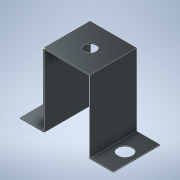
# Autodesk Inventor part: cla3
Saved by Autodesk Inventor 2021 (Build 250183000, 183)
## iProperties
Created: 2021-07-06
Part Number: cla3
Material: Iron, Cast
Document SubType Name: Modeling
Designer: KAVYA
Density: 7.15 g/cm^3
Appearance: Iron Gray
Author: KAVYA
Autodesk Inventor part; units mm, degrees
ref_plane "YZ Plane" through (0, 0, 0) normal (1, 0, 0) x (0, 1, 0)
ref_plane "XZ Plane" through (0, 0, 0) normal (0, 1, 0) x (-1, 0, 0)
ref_plane "XY Plane" through (0, 0, 0) normal (0, 0, 1) x (1, 0, 0)
sketch "Sketch1" plane through (0, 0, 0) normal (0, 1, 0) x (-1, 0, 0)
  line L0 (0, 0) -> (-48, 0)
  line L1 (-48, 0) -> (-48, -50)
  line L2 (-48, -50) -> (0, -50)
  line L3 (0, -50) -> (0, 0)
  dimension "d0" = 48
  dimension "d1" = 50
  constraints: 8 end point, 2 parallel, 1 horizontal, 1 perpendicular
  measures "d0" distance of L2.end L1.end
  measures "d1" distance of L1.end L0.end
extrude "Extrusion1" add sketch "Sketch1" along normal blind 1
sketch "Sketch2" plane through (48, 0, 0) normal (1, 0, 0) x (0, 0, -1)
  line L0 (0, 1) -> (50, 1) projected
  line L1 (0, 1) -> (50, 1)
  line L2 (50, 1) -> (50, -76)
  line L3 (50, -76) -> (0, -76)
  line L4 (0, -76) -> (0, 1)
  point P0 (0, 0)
  dimension "d4" = 50
  dimension "d5" = 77
  constraints: 8 end point, 2 parallel, 1 horizontal, 1 perpendicular
  measures "d4" distance of L2.end L3.end
  measures "d5" distance of L1.end L2.end
extrude "Extrusion2" add sketch "Sketch2" along normal blind 1
sketch "Sketch3" plane through (0, 0, -50) normal (-1, 0, 0) x (0, 0, 1)
  line L0 (0, 0) -> (0, 1) projected
  line L1 (50, 0) -> (50, -76) projected
  line L2 (0, 1) -> (50, 1)
  line L3 (50, 1) -> (50, -76)
  line L4 (50, -76) -> (0, -76)
  line L5 (0, -76) -> (0, 1)
  constraints: 8 end point, 2 parallel, 1 horizontal, 1 perpendicular
extrude "Extrusion3" add sketch "Sketch3" along normal blind 1
sketch "Sketch4" plane through (0, 1, 0) normal (0, 1, 0) x (1, 0, 0)
  point P0 (0, 0)
sketch "Sketch5" plane through (0, -76, -50) normal (0, -1, 0) x (1, 0, 0)
  line L0 (0, 50) -> (-26, 50)
  line L1 (-26, 50) -> (-26, 0)
  line L2 (-26, 0) -> (0, 0)
  line L3 (0, 0) -> (0, 50)
  line L4 (48, 50) -> (48, 0) projected
  line L5 (48, 50) -> (74, 50)
  line L6 (74, 50) -> (74, 0)
  line L7 (74, 0) -> (48, 0)
  line L8 (48, 0) -> (48, 50)
  dimension "d10" = 26
  dimension "d11" = 26
  constraints: 16 end point, 4 parallel, 2 horizontal, 2 perpendicular
  measures "d10" distance of L2.end L1.end
  measures "d11" distance of L6.end L7.end
extrude "Extrusion4" add sketch "Sketch5" along normal blind 1
sketch "Sketch6" plane through (0, 1, 0) normal (0, 1, 0) x (1, 0, 0)
  circle A0 centre (24, 25) radius 6.5
  line L0 (-1, 50) -> (49, 50) projected
  line L1 (49, 50) -> (49, 0) projected
  line L2 (49, 50) -> (74, 50) projected
  line L3 (74, 50) -> (74, 0) projected
  line L4 (-26, 50) -> (-1, 50) projected
  line L5 (-26, 0) -> (-26, 50) projected
  point P0 (0, 0)
  dimension "d14" = 13
  dimension "d17" = 25
  dimension "d18" = 25
  constraints: 1 centre point
  measures "d14" diameter of A0
  measures "d17" distance from line of L0 A0.centre
  measures "d18" distance from line of L1 A0.centre
extrude "Extrusion5" cut sketch "Sketch6" against normal blind 1
sketch "Sketch7" plane through (0, -76, -50) normal (0, 1, 0) x (1, 0, 0)
  circle A0 centre (61.5, -25) radius 7.75
  circle A1 centre (-13.5, -25) radius 7.75
  line L0 (-26, 0) -> (-1, 0) projected
  line L1 (-26, -50) -> (-26, 0) projected
  line L2 (74, 0) -> (74, -50) projected
  line L3 (49, 0) -> (74, 0) projected
  point P0 (0, -50)
  dimension "d25" = 15.5
  dimension "d26" = 15.5
  dimension "d27" = 25
  dimension "d28" = 12.5
  dimension "d29" = 12.5
  dimension "d30" = 25
  constraints: 2 centre point
  measures "d25" diameter of A0
  measures "d26" diameter of A1
  measures "d27" distance from line of L0 A1.centre
  measures "d28" distance from line of L1 A1.centre
  measures "d29" distance from line of L2 A0.centre
  measures "d30" distance from line of L3 A0.centre
extrude "Extrusion6" cut sketch "Sketch7" against normal blind 15.5
equation "\"d31\" = d25"
body "Solid1"
